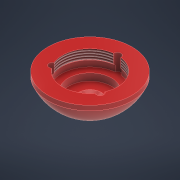
# Autodesk Inventor part: 015
Saved by Autodesk Inventor 2022 (Build 260153000, 153)
## iProperties
Created: 2021-11-02
Part Number: 015
Material: Stainless Steel, Austenitic
Document SubType Name: Modeling
Designer: vinicius.miguel
Density: 8 g/cm^3
Appearance: Red
Mass: 36.4387 g
Surface Area: 33.5564 cm^2
Volume: 4.55483 cm^3
Author: vinicius.miguel
Autodesk Inventor part; units mm, degrees
ref_plane "YZ Plane" through (0, 0, 0) normal (1, 0, 0) x (0, 1, 0)
ref_plane "XZ Plane" through (0, 0, 0) normal (0, 1, 0) x (-1, 0, 0)
ref_plane "XY Plane" through (0, 0, 0) normal (0, 0, 1) x (1, 0, 0)
sketch "Sketch1" plane through (0, 0, 0) normal (0, 0, 1) x (1, 0, 0)
  line L0 (-35.8694, 36.1667) -> (26.1213, 35.095) construction
  line L1 (26.1213, 35.095) -> (24.9917, -30.2436) construction
  line L2 (24.9917, -30.2436) -> (-36.999, -29.1719) construction
  line L3 (-36.999, -29.1719) -> (-35.8694, 36.1667) construction
  line L4 (0, -29.8115) -> (0, 35.5466) construction
  line L5 (-17.5, 14) -> (17.5, 14)
  line L6 (17.5, 14) -> (17.5, 12)
  arc A0 (0, 0.1813) -> (17.5, 12) centre (-0.0907, 19.1811) ccw
  arc A1 (1.5, 2.169) -> (2.1161, 0.3097) centre (2, 1.3029) ccw
  line L7 (12, 7) -> (12, 9.5)
  line L8 (12, 9.5) -> (11, 10.5)
  line L9 (11, 10.5) -> (11, 14)
  line L10 (4.6714, 4) -> (9, 4)
  line L11 (9, 4) -> (9, 7)
  line L12 (9, 7) -> (12, 7)
  line L13 (1.5, 2.169) -> (4.6714, 4)
  line L14 (1.5, 2.169) -> (0, 1.3029)
  point P0 (0, 0)
  point P1 (0, 14)
  point P2 (0, 0)
  dimension "d3" = 26.1213
  dimension "d7" = 24.9955
  dimension "d9" = 35
  dimension "d10" = 62
  dimension "d18" = 21.5466
  dimension "d19" = 14
  dimension "d26" = 19
  dimension "d27" = 1
  dimension "d34" = 22
  dimension "d38" = 135
  dimension "d39" = 2
  dimension "d41" = 2
  dimension "d44" = 24
  dimension "d54" = 11.831
  dimension "d82" = 18
  dimension "d83" = 10
  dimension "d86" = 7
  dimension "d87" = 3.5
  dimension "d90" = 150
  constraints: 22 end point, 7 point on line, 5 point on circle, 3 perpendicular, 2 centre point, 2 tangent, 1 coincident, 1 collinear, 1 horizontal, 1 midpoint, 1 parallel, 1 vertical, 1 vertical alignment, 2 other
  measures "d3" distance from line of L0.end L4
  measures "d7" distance of L1.end L4.start
  measures "d9" distance of L5.start L5.end
  measures "d10" distance of L0.start L0.end
  measures "d18" distance from line of L4.end L5
  measures "d19" distance of point (0, 14) point (0, 0)
  measures "d26" radius of A0
  measures "d27" radius of A1
  measures "d34" diameter of L9 L4
  measures "d38" angle of L7 L8
  measures "d39" distance centre to line of A1 L4
  measures "d41" distance of L5.end L6.end
  measures "d44" diameter of L7 L4
  measures "d54" vertical distance of point (0, 14) L13.start
  measures "d82" diameter of L11 L4
  measures "d83" distance between parallel lines of L5 L10
  measures "d86" distance between parallel lines of L5 L12
  measures "d87" distance of L8.end L9.end
  measures "d90" angle of L10 L13
revolve "Revolution1" add sketch "Sketch1" angle 360 about axis through (0, -29.8115, 0) along (0, 1, 0)
sketch "Sketch2" plane through (0, 14, 0) normal (0, 1, 0) x (1, 0, 0)
  circle A0 centre (0, 0) radius 11 projected
  point P0 (0, 0)
  constraints: 1 coincident
hole "Hole1" at (0, 14, 0) direction (0, -1, 0) diameter 22.9175 depth 5 thread size "M24x1" class "6H" standard "ISO Metric profile"
sketch "Sketch3" plane through (0, 14, 0) normal (0, 1, 0) x (1, 0, 0)
  circle A0 centre (0, 0) radius 11.4587 projected
  point P0 (0, 0)
  point P1 (0, 11.4587)
  constraints: 2 vertical alignment, 1 other
hole "Hole2" at (0, 14, -11.4587) direction (0, -1, 0) diameter 3 depth 7
pattern_circular "Circular Pattern1" count 3 over 360 about axis through (0, 13, 0) along (0, -1, 0) of "Hole2"
equation "\"d3\" = 0.421311 * d10"
equation "\"d7\" = 0.403153 * d10"
equation "\"d18\" = 0.347525 * d10"
body "Solid1"
